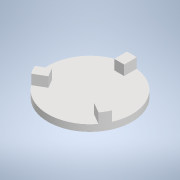
# Autodesk Inventor part: PM Base
Saved by Autodesk Inventor 2021 (Build 250183000, 183)
## iProperties
Created: 2021-05-05
Part Number: PM Base
Material: Generic
Document SubType Name: Modeling
Designer: techv
Density: 1 g/cm^3
Appearance: Default
Author: techv
Autodesk Inventor part; units mm, degrees
ref_plane "YZ Plane" through (0, 0, 0) normal (1, 0, 0) x (0, 1, 0)
ref_plane "XZ Plane" through (0, 0, 0) normal (0, 1, 0) x (-1, 0, 0)
ref_plane "XY Plane" through (0, 0, 0) normal (0, 0, 1) x (1, 0, 0)
sketch "Sketch1" plane through (0, 0, 0) normal (0, 1, 0) x (-1, 0, 0)
  circle A0 centre (0, 0) radius 63.5
  dimension "d0" = 127
  constraints: 1 centre point, 1 coincident
  measures "d0" diameter of A0
extrude "Extrusion1" add sketch "Sketch1" along normal blind 10
sketch "Sketch2" plane through (0, 10, 0) normal (0, 1, 0) x (1, 0, 0)
  line L0 (0, 0) -> (0, 63.7295)
  circle A0 centre (0, 0) radius 63.5 projected
  line L1 (7.5, 44.1365) -> (-7.5, 44.1365)
  line L2 (-7.5, 44.1365) -> (-7.5, 64.1365)
  line L3 (-7.5, 64.1365) -> (7.5, 64.1365)
  line L4 (7.5, 64.1365) -> (7.5, 44.1365)
  line L5 (7.5, 44.1365) -> (-7.5, 64.1365) construction
  line L6 (-7.5, 44.1365) -> (7.5, 64.1365) construction
  point P0 (0, 54.1365)
  point P1 (-7.5, 63.0555)
  point P2 (7.5, 63.0555)
  dimension "d3" = 15
  dimension "d4" = 20
  constraints: 14 end point, 2 midpoint, 2 parallel, 1 horizontal, 1 perpendicular, 1 point on line, 1 vertical
  measures "d3" distance of L2.end L3.end
  measures "d4" distance of L1.end L2.end
extrude "Extrusion2" add sketch "Sketch2" along normal blind 15 contours L1 L2 A0 L0 | L0 A0 L4 L1
pattern_circular "Circular Pattern1" count 3 over 360 about axis through (0, 0, 0) along (0, 1, 0) of "Extrusion2"
sketch "Sketch3" plane through (0, 0, 0) normal (0, -1, 0) x (1, 0, 0)
  circle A0 centre (0, 0) radius 15
  dimension "d10" = 30
  constraints: 1 centre point, 1 coincident
  measures "d10" diameter of A0
extrude "Extrusion3" add sketch "Sketch3" along normal blind 5
body "Solid1"
